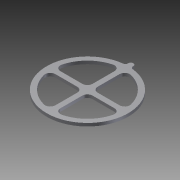
# Autodesk Inventor part: OpenROV 2_2 Prop Guard
Saved by Autodesk Inventor 2011 (Build 150239000, 239)
## iProperties
Created: 2011-11-07
Part Number: OpenROV 2_2 Prop Guard
Document SubType Name: Modeling
Designer: user
Density: 1 g/cm^3
Author: user
Autodesk Inventor part; units mm, degrees
ref_plane "YZ Plane" through (0, 0, 0) normal (1, 0, 0) x (0, 1, 0)
ref_plane "XZ Plane" through (0, 0, 0) normal (0, 1, 0) x (-1, 0, 0)
ref_plane "XY Plane" through (0, 0, 0) normal (0, 0, 1) x (1, 0, 0)
sketch "Sketch1" plane through (0, 0, 0) normal (0, 0, 1) x (1, 0, 0)
  line L0 (39.9382, 2.7778) -> (39.9382, -2.2222)
  line L1 (-39.9382, -2.7778) -> (-39.9382, 2.2222)
  arc A0 (33.8886, 8.75) -> (8.75, 33.8886) centre (0, 0) ccw
  arc A1 (8.75, -33.8886) -> (33.8886, -8.75) centre (0, 0) ccw
  arc A2 (-8.75, 33.8886) -> (-33.8886, 8.75) centre (0, 0) ccw
  arc A3 (-33.8886, -8.75) -> (-8.75, -33.8886) centre (0, 0) ccw
  line L2 (2.5, 29.0474) -> (2.5, 7.5)
  line L3 (2.5, -7.5) -> (2.5, -29.0474)
  line L4 (-29.0474, 2.5) -> (-7.5, 2.5)
  line L5 (7.5, 2.5) -> (29.0474, 2.5)
  line L6 (-2.5, -29.0474) -> (-2.5, -7.5)
  line L7 (-2.5, 7.5) -> (-2.5, 29.0474)
  line L8 (29.0474, -2.5) -> (7.5, -2.5)
  line L9 (-7.5, -2.5) -> (-29.0474, -2.5)
  arc A4 (-2.5, 29.0474) -> (-8.75, 33.8886) centre (-7.5, 29.0474) ccw
  arc A5 (8.75, 33.8886) -> (2.5, 29.0474) centre (7.5, 29.0474) ccw
  arc A6 (29.0474, 2.5) -> (33.8886, 8.75) centre (29.0474, 7.5) ccw
  arc A7 (33.8886, -8.75) -> (29.0474, -2.5) centre (29.0474, -7.5) ccw
  arc A8 (2.5, -29.0474) -> (8.75, -33.8886) centre (7.5, -29.0474) ccw
  arc A9 (-8.75, -33.8886) -> (-2.5, -29.0474) centre (-7.5, -29.0474) ccw
  arc A10 (-29.0474, -2.5) -> (-33.8886, -8.75) centre (-29.0474, -7.5) ccw
  arc A11 (-33.8886, 8.75) -> (-29.0474, 2.5) centre (-29.0474, 7.5) ccw
  arc A12 (-7.5, 2.5) -> (-2.5, 7.5) centre (-7.5, 7.5) ccw
  arc A13 (2.5, 7.5) -> (7.5, 2.5) centre (7.5, 7.5) ccw
  arc A14 (7.5, -2.5) -> (2.5, -7.5) centre (7.5, -7.5) ccw
  arc A15 (-2.5, -7.5) -> (-7.5, -2.5) centre (-7.5, -7.5) ccw
  arc A16 (-4.7059, 39.7222) -> (4.7059, 39.7222) centre (0, 0) ccw
  line L10 (0, 45) -> (0, 45)
  line L11 (2.5, 42.5) -> (2.5, 42.2049)
  line L12 (-2.5, 26.931) -> (-2.5, 29.0474)
  line L13 (-2.5, 42.2049) -> (-2.5, 42.5)
  arc A17 (-4.7059, 39.7222) -> (-2.5, 42.2049) centre (-5, 42.2049) ccw
  arc A18 (0, 45) -> (-2.5, 42.5) centre (0, 42.5) ccw
  arc A19 (2.5, 42.5) -> (0, 45) centre (0, 42.5) ccw
  arc A20 (2.5, 42.2049) -> (4.7059, 39.7222) centre (5, 42.2049) ccw
  point P0 (-2.5, 34.9106)
  point P1 (2.5, 34.9106)
  point P2 (34.9106, 2.5)
  point P3 (34.9106, -2.5)
  point P4 (2.5, -34.9106)
  point P5 (-2.5, -34.9106)
  point P6 (-34.9106, -2.5)
  point P7 (-34.9106, 2.5)
  point P8 (-2.5, 39.9218)
  point P9 (2.5, 39.9218)
  dimension "d6" = 5
  dimension "d7" = 5
  dimension "d8" = 5
  dimension "d9" = 5
  dimension "d10" = 35
  dimension "d11" = 35
  dimension "d12" = 35
  dimension "d13" = 35
  dimension "d14" = 2.5
  dimension "d15" = 2.5
  dimension "d16" = 2.5
  dimension "d17" = 2.5
  dimension "d18" = 5
  dimension "d24" = 80
  dimension "d25" = 45
  dimension "d26" = 2.5
  constraints: 52 point on circle, 33 tangent, 28 end point, 21 centre point, 14 equal radius, 11 parallel, 11 point on line, 6 perpendicular, 2 horizontal, 1 coincident
  measures "d6" distance between parallel lines of L2 L7
  measures "d7" distance between parallel lines of L8 L5
  measures "d8" distance between parallel lines of L6 L3
  measures "d9" distance between parallel lines of L9 L4
  measures "d10" radius of A2
  measures "d11" radius of A0
  measures "d12" radius of A1
  measures "d13" radius of A3
  measures "d14" distance from line of L4 point (0, 0)
  measures "d15" distance from line of L2 point (0, 0)
  measures "d16" distance from line of L8 point (0, 0)
  measures "d17" distance from line of L6 point (0, 0)
  measures "d18" radius of A4
  measures "d24" diameter of A16
  measures "d25" distance from line of point (0, 0) L10
  measures "d26" radius of A17
extrude "Extrusion2" add sketch "Sketch1" along normal blind 3
body "Solid2"
